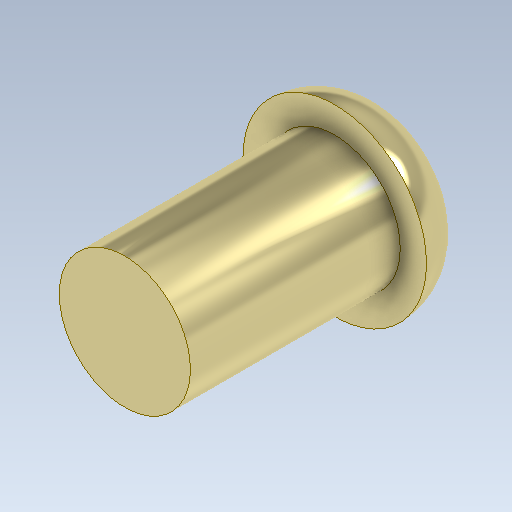
# Autodesk Inventor part: surub ochelari
Saved by Autodesk Inventor 2020 (Build 240168000, 168)
## iProperties
Created: 2019-11-27
Part Number: surub ochelari
Material: Iron, Cast
Document SubType Name: Modeling
Designer: Bianca
Density: 7.15 g/cm^3
Appearance: Iron Gray
Mass: 0.00360368 g
Surface Area: 0.141224 cm^2
Volume: 0.0033997 cm^3
Author: Bianca
Autodesk Inventor part; units mm, degrees
ref_plane "YZ Plane" through (0, 0, 0) normal (1, 0, 0) x (0, 1, 0)
ref_plane "XZ Plane" through (0, 0, 0) normal (0, 1, 0) x (-1, 0, 0)
ref_plane "XY Plane" through (0, 0, 0) normal (0, 0, 1) x (1, 0, 0)
sketch "Sketch1" plane through (0, 0, 0) normal (0, 0, 1) x (1, 0, 0)
  circle A0 centre (0, 0) radius 0.625
  circle A1 centre (0, 0) radius 0.75
  dimension "d0" = 1.25
  dimension "d3" = 1.5
  constraints: 2 centre point, 2 coincident
  measures "d0" diameter of A0
  measures "d3" diameter of A1
extrude "Extrusion1" add sketch "Sketch1" along normal blind 2 contours A0
sketch "Sketch2" plane through (0, 0, 0) normal (0, 0, -1) x (-1, 0, 0)
  circle A0 centre (0, 0) radius 0.875
  dimension "d4" = 1.75
  constraints: 1 centre point, 1 coincident
  measures "d4" diameter of A0
extrude "Extrusion2" add sketch "Sketch2" along normal blind 0.5
fillet "Fillet1" radius 0.5 1 edges at (0.875, 0, -0.5)
sketch "Sketch3" plane through (0, 0, 0) normal (1, 0, 0) x (0, 1, 0)
  point P0 (0, 0)
body "Solid1"
